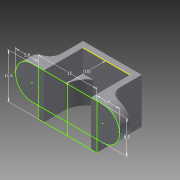
# Autodesk Inventor part: Motor_Bracket
Saved by Autodesk Inventor 2015 (Build 190159000, 159)
## iProperties
Created: 2014-10-28
Part Number: Motor_Bracket
Material: Generic
Document SubType Name: Modeling
Designer: s4201025
Density: 1 g/cm^3
Appearance: Default
Author: s4201025
Autodesk Inventor part; units mm, degrees
ref_plane "YZ Plane" through (0, 0, 0) normal (1, 0, 0) x (0, 1, 0)
ref_plane "XZ Plane" through (0, 0, 0) normal (0, 1, 0) x (-1, 0, 0)
ref_plane "XY Plane" through (0, 0, 0) normal (0, 0, 1) x (1, 0, 0)
sketch "Sketch1" plane through (0, 0, 0) normal (0, 1, 0) x (-1, 0, 0)
  line L0 (-7.55, 0) -> (0, 0)
  line L1 (0, -11.5) -> (-7.5, -11.5)
  line L2 (-7.5, 0) -> (-9.05, 0)
  line L3 (-9.05, -8.5) -> (0, -8.5)
  arc A0 (-9.05, 0) -> (-9.05, -8.5) centre (-9.05, -4.25) ccw
  line L4 (-7.55, 0) -> (-7.3, 0)
  line L5 (-7.3, -11.5) -> (-7.5, -11.5)
  line L6 (-7.55, 0) -> (-7.5, 0)
  line L7 (-7.5, -11.5) -> (-7.5, -11.5)
  line L8 (0, 0) -> (0, -11.5)
  line L9 (-7.5, 0) -> (-7.5, -8.5)
  line L10 (7.55, 0) -> (0, 0)
  line L11 (0, -11.5) -> (7.55, -11.5)
  line L12 (7.5, 0) -> (9.05, 0)
  line L13 (9.05, -8.5) -> (0, -8.5)
  arc A1 (9.05, -8.5) -> (9.05, 0) centre (9.05, -4.25) ccw
  line L14 (7.55, 0) -> (7.3, 0)
  line L15 (7.3, -11.5) -> (7.55, -11.5)
  line L16 (7.55, 0) -> (7.5, 0)
  line L17 (7.5, -11.5) -> (7.5, -11.5)
  line L18 (7.5, 0) -> (7.5, -11.5)
  line L19 (7.5, 0) -> (-7.5, 0)
  line L20 (-7.5, 0) -> (-7.5, -11.5)
  line L21 (-7.5, -11.5) -> (7.5, -11.5)
  line L22 (7.5, -11.5) -> (7.5, 0)
  line L23 (-7.5, -8.5) -> (-7.5, -11.5)
  point P0 (0, 0)
  point P1 (-7.55, -8.5)
  point P2 (-13.3, -4.25)
  point P3 (7.55, -8.5)
  point P4 (13.3, -4.25)
  point P5 (7.5, -8.5)
  dimension "d3" = 8.5
  dimension "d9" = 5.8
  dimension "d25" = 15
  dimension "d26" = 5.8
  dimension "d27" = 11.5
  constraints: 48 end point, 13 point on line, 11 symmetric about line, 8 parallel, 5 horizontal, 5 point on circle, 2 centre point, 2 perpendicular, 1 other
  measures "d3" distance of L3.start L2.end
  measures "d9" distance from line of L9 point (-13.3, -4.25)
  measures "d25" distance between parallel lines of L22 L9
  measures "d27" distance between parallel lines of L10 L11
extrude "Extrusion1" add sketch "Sketch1" along normal blind 11.5 contours L0 L8 L3 L9 | L3 L8 L1 L20 | L10 L18 L13 L8 | L13 L18 L11 L8
sketch "Sketch2" plane through (-7.5, 0, 0) normal (0, 0, 1) x (1, 0, 0)
  line L0 (0, 0) -> (15, 0) projected
  line L1 (1, 0) -> (14, 0)
  line L2 (0, 11.5) -> (15, 11.5) projected
  line L3 (1.5, 0) -> (13.5, 0)
  line L4 (13.5, 0) -> (13.5, 10)
  line L5 (13.5, 10) -> (1.5, 10)
  line L6 (1.5, 10) -> (1.5, 0)
  point P0 (7.5, 0)
  point P1 (14, 10.5)
  point P2 (1, 10.5)
  dimension "d14" = 10.5
  dimension "d28" = 11.5
  dimension "d29" = 12
  dimension "d30" = 10
  constraints: 10 end point, 2 horizontal, 2 parallel, 2 point on line, 1 perpendicular
  measures "d14" distance of point (14, 10.5) L1.end
  measures "d28" distance between parallel lines of L0 L2
  measures "d29" distance of L5.end L4.end
  measures "d30" distance of L4.end L3.end
extrude "Extrusion3" add sketch "Sketch1" along normal blind 3 contours L0 L9 L3 A0 L2
extrude "Extrusion4" add sketch "Sketch1" along normal blind 3 contours L18 L10 L12 A1 L13
fillet "Fillet1" radius 3 1 edges at (-7.5, 3, -4.25)
fillet "Fillet2" radius 3 1 edges at (7.5, 3, -4.25)
extrude "Extrusion5" cut sketch "Sketch2" against normal blind 5.75
sketch "Sketch3" plane through (7.5, 0, -11.5) normal (0, 0, -1) x (-1, 0, 0)
  line L0 (1.5, 0) -> (13.5, 0)
  line L1 (13.5, 0) -> (13.5, 5)
  line L2 (10.8166, 10) -> (4.1834, 10)
  line L3 (1.5, 5) -> (1.5, 0)
  arc A0 (4.1834, 10) -> (1.5, 5) centre (7.5, 5) ccw
  arc A1 (13.5, 5) -> (10.8166, 10) centre (7.5, 5) ccw
  point P0 (7.5, 0)
  point P1 (13.5, 10)
  point P2 (1.5, 10)
  dimension "d33" = 12
  dimension "d34" = 10
  constraints: 8 end point, 4 point on circle, 4 point on line, 2 centre point, 2 parallel, 1 horizontal, 1 perpendicular
  measures "d33" distance of point (1.5, 10) point (13.5, 10)
  measures "d34" distance of point (13.5, 10) L0.end
extrude "Extrusion6" cut sketch "Sketch3" against normal blind 5.75
sketch "Sketch4" plane through (-7.5, 11.5, 0) normal (0, 0, 1) x (1, 0, 0)
  line L0 (1.5, -1.5) -> (13.5, -1.5) projected
  point P0 (7.5, -11.5)
  dimension "d40" = 10
  measures "d40" distance from line of point (7.5, -11.5) L0
body "Solid1"
